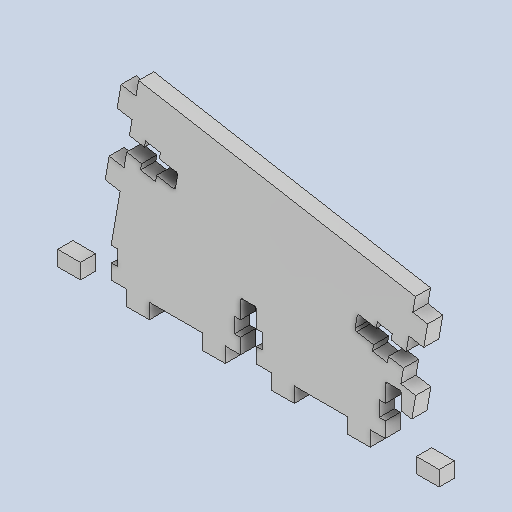
# Autodesk Inventor part: tc_support_down
Saved by Autodesk Inventor 2024.1 (Build 281209000, 209)
## iProperties
Created: 2019-07-16
Part Number: tc_support_down
Material: Acier inoxydable
Document SubType Name: Modeling
Designer: Thibault
Density: 8 g/cm^3
Appearance: Semi-poli
extra_height_front: 10,900 mm
extra_height_back: 4,367 mm
tc_base_support_dist: 37,050 mm
tc_anchor_dist: 19,100 mm
Author: Thibault
Autodesk Inventor part; units mm, degrees
ref_plane "YZ Plane" through (0, 0, 0) normal (1, 0, 0) x (0, 1, 0)
ref_plane "XZ Plane" through (0, 0, 0) normal (0, 1, 0) x (-1, 0, 0)
ref_plane "XY Plane" through (0, 0, 0) normal (0, 0, 1) x (1, 0, 0)
sketch "Anchor (nut side)" plane through (0, 0, 0) normal (0, 0, 1) x (1, 0, 0)
  line L0 (11.1, 0) -> (9.1, 0)
  line L1 (9.1, 0) -> (9.1, -2)
  line L2 (9.1, -2) -> (9.9, -2)
  line L3 (9.9, -2) -> (9.9, -4)
  line L4 (6.2, -4) -> (6.2, -2)
  line L5 (6.2, -2) -> (7, -2)
  line L6 (7, -2) -> (7, 0)
  line L7 (7, 0) -> (5, 0)
  line L8 (2, 0) -> (2, 2)
  line L9 (2, 0) -> (3, 0) construction
  line L10 (2, 2) -> (5, 2)
  line L11 (5, 2) -> (5, 0)
  line L12 (11.1, 0) -> (11.1, 2)
  line L13 (11.1, 2) -> (14.1, 2)
  line L14 (14.1, 2) -> (14.1, 0)
  line L15 (0, 0) -> (2, 0)
  line L16 (14.1, 0) -> (16.1, 0)
  line L17 (6.2, -4) -> (7, -4)
  line L18 (9.9, -4) -> (9.1, -4)
  line L19 (7, -4) -> (7, -6.25)
  line L20 (9.1, -4) -> (9.1, -6.25)
  line L21 (7.25, -6.5) -> (8.05, -6.5)
  arc A0 (7, -6.25) -> (7.25, -6.5) centre (7.25, -6.25) ccw
  arc A1 (8.85, -6.5) -> (9.1, -6.25) centre (8.85, -6.25) ccw
  line L22 (8.05, -6.5) -> (8.85, -6.5)
  line L23 (8.05, -3.8983) -> (8.05, -9.959) construction
  point P0 (9.1321, -0.6227)
  point P1 (7, -6.5)
  point P2 (9.1, -6.5)
  dimension "d3" = 2
  dimension "d7" = 6.1
  dimension "d10" = 2
  dimension "d11" = 2
  dimension "d12" = 0.8
  dimension "d13" = 2
  dimension "d14" = 0.8
  dimension "d15" = 2.1
  dimension "d18" = 2
  dimension "d19" = 0.8
  dimension "d20" = 0.8
  dimension "d21" = 2.5
  dimension "d22" = 2.5
  dimension "d23" = 2.1
  dimension "d38" = 2
  dimension "d39" = 0.25
  dimension "d120" = 3
  measures "d3" distance of point (0, 0) L8.start
  measures "d7" distance of L7.end L0.start
  measures "d10" distance of L0.start L0.end
  measures "d11" distance of L0.end L1.end
  measures "d12" distance of L1.end L2.end
  measures "d13" distance of L2.end L3.end
  measures "d14" distance of L4.end L5.end
  measures "d15" distance of L6.end L0.end
  measures "d18" distance of L14.end point (16.1, 0)
  measures "d19" distance of L4.start L17.end
  measures "d20" distance of L3.end L18.end
  measures "d21" distance of L17.end point (7, -6.5)
  measures "d22" distance of L18.end point (9.1, -6.5)
  measures "d23" distance of L17.end L18.end
  measures "d38" distance of the line from the sketch origin of L10
  measures "d39" radius of A0
  measures "d120" distance of L8.end L10.end
sketch "Anchor (screw side)" plane through (0, 0, 0) normal (0, 0, 1) x (1, 0, 0)
  circle A0 centre (93.8994, 50.2542) radius 1.05
  line L0 (90.8494, 51.2542) -> (87.8494, 51.2542)
  line L1 (87.8494, 51.2542) -> (87.8494, 49.2542)
  line L2 (87.8494, 49.2542) -> (90.8494, 49.2542)
  line L3 (90.8494, 49.2542) -> (90.8494, 51.2542)
  line L4 (99.9494, 51.2542) -> (96.9494, 51.2542)
  line L5 (96.9494, 51.2542) -> (96.9494, 49.2542)
  line L6 (96.9494, 49.2542) -> (99.9494, 49.2542)
  line L7 (99.9494, 49.2542) -> (99.9494, 51.2542)
  line L8 (90.8494, 51.2542) -> (96.9494, 49.2542) construction
  line L9 (96.9494, 51.2542) -> (90.8494, 49.2542) construction
  line L10 (85.8494, 53.2542) -> (101.9494, 53.2542) construction
  line L11 (101.9494, 53.2542) -> (101.9494, 47.2542) construction
  line L12 (101.9494, 47.2542) -> (85.8494, 47.2542) construction
  line L13 (85.8494, 47.2542) -> (85.8494, 53.2542) construction
  point P0 (103.5798, 50.1132)
  dimension "d27" = 2.1
  dimension "d28" = 3
  dimension "d29" = 2
  dimension "slot_distance" = 6.1
  dimension "d34" = 2
  dimension "d35" = 2
  dimension "d36" = 2
  dimension "d37" = 2
  measures "d27" diameter of A0
  measures "d28" distance of L2.end L1.end
  measures "d29" distance of L1.end L0.end
  measures "slot_distance" distance between parallel lines of L5 L3
  measures "d34" distance between parallel lines of L0 L10
  measures "d35" distance between parallel lines of L12 L2
  measures "d36" distance between parallel lines of L11 L7
  measures "d37" distance between parallel lines of L13 L1
derived "shared_parameters.ipt"
sketch "Esquisse2" plane through (0, 0, 0) normal (0, 0, 1) x (1, 0, 0)
  line L0 (-1.0016, 15.2398) -> (1.9984, 15.2398)
  line L1 (18.0984, 15.2398) -> (21.0984, 15.2398)
  line L2 (-17.1016, 15.2398) -> (-8.7624, 15.2398)
  line L3 (37.1984, 15.2398) -> (28.8592, 15.2398)
  line L4 (-8.7624, 15.2398) -> (-7.2169, 24.0046)
  line L5 (-4.4212, 39.86) -> (32.066, 33.4264)
  line L6 (29.2702, 17.571) -> (28.8592, 15.2398)
  line L7 (-12.1016, 15.2398) -> (-10.1016, 15.2398)
  line L8 (-10.1016, 15.2398) -> (-10.1016, 17.2398)
  line L9 (-10.1016, 17.2398) -> (-10.9016, 17.2398)
  line L10 (-10.9016, 17.2398) -> (-10.9016, 19.2398)
  line L11 (-7.2016, 19.2398) -> (-7.2016, 17.2398)
  line L12 (-7.2016, 17.2398) -> (-8.0016, 17.2398)
  line L13 (-8.0016, 17.2398) -> (-8.0016, 15.2398)
  line L14 (-8.0016, 15.2398) -> (-6.0016, 15.2398)
  line L15 (-3.0016, 15.2398) -> (-3.0016, 13.2398)
  line L16 (-3.0016, 15.2398) -> (-4.0016, 15.2398) construction
  line L17 (-3.0016, 13.2398) -> (-6.0016, 13.2398)
  line L18 (-6.0016, 13.2398) -> (-6.0016, 15.2398)
  line L19 (-12.1016, 15.2398) -> (-12.1016, 13.2398)
  line L20 (-12.1016, 13.2398) -> (-15.1016, 13.2398)
  line L21 (-15.1016, 13.2398) -> (-15.1016, 15.2398)
  line L22 (-1.0016, 15.2398) -> (-3.0016, 15.2398)
  line L23 (-15.1016, 15.2398) -> (-17.1016, 15.2398)
  line L24 (-7.2016, 19.2398) -> (-8.0016, 19.2398)
  line L25 (-10.9016, 19.2398) -> (-10.1016, 19.2398)
  line L26 (-8.0016, 19.2398) -> (-8.0016, 21.4898)
  line L27 (-10.1016, 19.2398) -> (-10.1016, 21.4898)
  line L28 (-8.2516, 21.7398) -> (-9.0516, 21.7398)
  arc A0 (-8.0016, 21.4898) -> (-8.2516, 21.7398) centre (-8.2516, 21.4898) ccw
  arc A1 (-9.8516, 21.7398) -> (-10.1016, 21.4898) centre (-9.8516, 21.4898) ccw
  line L29 (-9.0516, 21.7398) -> (-9.8516, 21.7398)
  line L30 (-9.0516, 19.1381) -> (-9.0516, 25.1989) construction
  line L31 (6.9984, 15.2398) -> (8.9984, 15.2398)
  line L32 (8.9984, 15.2398) -> (8.9984, 17.2398)
  line L33 (8.9984, 17.2398) -> (8.1984, 17.2398)
  line L34 (8.1984, 17.2398) -> (8.1984, 19.2398)
  line L35 (11.8984, 19.2398) -> (11.8984, 17.2398)
  line L36 (11.8984, 17.2398) -> (11.0984, 17.2398)
  line L37 (11.0984, 17.2398) -> (11.0984, 15.2398)
  line L38 (11.0984, 15.2398) -> (13.0984, 15.2398)
  line L39 (16.0984, 15.2398) -> (16.0984, 13.2398)
  line L40 (16.0984, 15.2398) -> (15.0984, 15.2398) construction
  line L41 (16.0984, 13.2398) -> (13.0984, 13.2398)
  line L42 (13.0984, 13.2398) -> (13.0984, 15.2398)
  line L43 (6.9984, 15.2398) -> (6.9984, 13.2398)
  line L44 (6.9984, 13.2398) -> (3.9984, 13.2398)
  line L45 (3.9984, 13.2398) -> (3.9984, 15.2398)
  line L46 (18.0984, 15.2398) -> (16.0984, 15.2398)
  line L47 (3.9984, 15.2398) -> (1.9984, 15.2398)
  line L48 (11.8984, 19.2398) -> (11.0984, 19.2398)
  line L49 (8.1984, 19.2398) -> (8.9984, 19.2398)
  line L50 (11.0984, 19.2398) -> (11.0984, 21.4898)
  line L51 (8.9984, 19.2398) -> (8.9984, 21.4898)
  line L52 (10.8484, 21.7398) -> (10.0484, 21.7398)
  arc A2 (11.0984, 21.4898) -> (10.8484, 21.7398) centre (10.8484, 21.4898) ccw
  arc A3 (9.2484, 21.7398) -> (8.9984, 21.4898) centre (9.2484, 21.4898) ccw
  line L53 (10.0484, 21.7398) -> (9.2484, 21.7398)
  line L54 (10.0484, 19.1381) -> (10.0484, 25.1989) construction
  line L55 (26.0984, 15.2398) -> (28.0984, 15.2398)
  line L56 (28.0984, 15.2398) -> (28.0984, 17.2398)
  line L57 (28.0984, 17.2398) -> (27.2984, 17.2398)
  line L58 (27.2984, 17.2398) -> (27.2984, 19.2398)
  line L59 (30.9984, 19.2398) -> (30.9984, 17.2398)
  line L60 (30.9984, 17.2398) -> (30.1984, 17.2398)
  line L61 (30.1984, 17.2398) -> (30.1984, 15.2398)
  line L62 (30.1984, 15.2398) -> (32.1984, 15.2398)
  line L63 (35.1984, 15.2398) -> (35.1984, 13.2398)
  line L64 (35.1984, 15.2398) -> (34.1984, 15.2398) construction
  line L65 (35.1984, 13.2398) -> (32.1984, 13.2398)
  line L66 (32.1984, 13.2398) -> (32.1984, 15.2398)
  line L67 (26.0984, 15.2398) -> (26.0984, 13.2398)
  line L68 (26.0984, 13.2398) -> (23.0984, 13.2398)
  line L69 (23.0984, 13.2398) -> (23.0984, 15.2398)
  line L70 (37.1984, 15.2398) -> (35.1984, 15.2398)
  line L71 (23.0984, 15.2398) -> (21.0984, 15.2398)
  line L72 (30.9984, 19.2398) -> (30.1984, 19.2398)
  line L73 (27.2984, 19.2398) -> (28.0984, 19.2398)
  line L74 (30.1984, 19.2398) -> (30.1984, 21.4898)
  line L75 (28.0984, 19.2398) -> (28.0984, 21.4898)
  line L76 (29.9484, 21.7398) -> (29.1484, 21.7398)
  arc A4 (30.1984, 21.4898) -> (29.9484, 21.7398) centre (29.9484, 21.4898) ccw
  arc A5 (28.3484, 21.7398) -> (28.0984, 21.4898) centre (28.3484, 21.4898) ccw
  line L77 (29.1484, 21.7398) -> (28.3484, 21.7398)
  line L78 (29.1484, 19.1381) -> (29.1484, 25.1989) construction
  line L79 (-5.2894, 34.936) -> (-5.6367, 32.9664)
  line L80 (-5.6367, 32.9664) -> (-3.6671, 32.6191)
  line L81 (-3.6671, 32.6191) -> (-3.5282, 33.4069)
  line L82 (-3.5282, 33.4069) -> (-1.5586, 33.0596)
  line L83 (-2.201, 29.4158) -> (-4.1707, 29.7631)
  line L84 (-4.1707, 29.7631) -> (-4.0317, 30.551)
  line L85 (-4.0317, 30.551) -> (-6.0014, 30.8983)
  line L86 (-6.0014, 30.8983) -> (-6.3487, 28.9287)
  line L87 (-6.8696, 25.9742) -> (-8.8392, 26.3215)
  line L88 (-6.8696, 25.9742) -> (-6.696, 26.9591) construction
  line L89 (-8.8392, 26.3215) -> (-8.3183, 29.276)
  line L90 (-8.3183, 29.276) -> (-6.3487, 28.9287)
  line L91 (-5.2894, 34.936) -> (-7.259, 35.2833)
  line L92 (-7.259, 35.2833) -> (-6.7381, 38.2377)
  line L93 (-6.7381, 38.2377) -> (-4.7685, 37.8904)
  line L94 (-7.2169, 24.0046) -> (-6.8696, 25.9742)
  line L95 (-4.7685, 37.8904) -> (-4.4212, 39.86)
  line L96 (-2.201, 29.4158) -> (-2.0621, 30.2037)
  line L97 (-1.5586, 33.0596) -> (-1.6975, 32.2718)
  line L98 (-2.0621, 30.2037) -> (0.1537, 29.813)
  line L99 (-1.6975, 32.2718) -> (0.5183, 31.8811)
  line L100 (0.4433, 30.0158) -> (0.5822, 30.8036)
  arc A6 (0.1537, 29.813) -> (0.4433, 30.0158) centre (0.1971, 30.0592) ccw
  arc A7 (0.7211, 31.5915) -> (0.5183, 31.8811) centre (0.4749, 31.6349) ccw
  line L101 (0.5822, 30.8036) -> (0.7211, 31.5915)
  line L102 (-1.98, 31.2554) -> (3.9887, 30.203) construction
  line L103 (30.1385, 22.495) -> (30.4858, 24.4646)
  line L104 (30.4858, 24.4646) -> (28.5162, 24.8119)
  line L105 (28.5162, 24.8119) -> (28.3772, 24.0241)
  line L106 (28.3772, 24.0241) -> (26.4076, 24.3714)
  line L107 (27.0501, 28.0152) -> (29.0197, 27.6679)
  line L108 (29.0197, 27.6679) -> (28.8808, 26.88)
  line L109 (28.8808, 26.88) -> (30.8504, 26.5327)
  line L110 (30.8504, 26.5327) -> (31.1977, 28.5023)
  line L111 (31.7187, 31.4568) -> (33.6883, 31.1095)
  line L112 (31.7187, 31.4568) -> (31.545, 30.4719) construction
  line L113 (33.6883, 31.1095) -> (33.1673, 28.155)
  line L114 (33.1673, 28.155) -> (31.1977, 28.5023)
  line L115 (30.1385, 22.495) -> (32.1081, 22.1477)
  line L116 (32.1081, 22.1477) -> (31.5871, 19.1933)
  line L117 (31.5871, 19.1933) -> (29.6175, 19.5406)
  line L118 (32.066, 33.4264) -> (31.7187, 31.4568)
  line L119 (29.6175, 19.5406) -> (29.2702, 17.571)
  line L120 (27.0501, 28.0152) -> (26.9112, 27.2273)
  line L121 (26.4076, 24.3714) -> (26.5465, 25.1592)
  line L122 (26.9112, 27.2273) -> (24.6954, 27.618)
  line L123 (26.5465, 25.1592) -> (24.3307, 25.5499)
  line L124 (24.4058, 27.4152) -> (24.2668, 26.6274)
  arc A8 (24.6954, 27.618) -> (24.4058, 27.4152) centre (24.652, 27.3718) ccw
  arc A9 (24.1279, 25.8395) -> (24.3307, 25.5499) centre (24.3741, 25.7961) ccw
  line L125 (24.2668, 26.6274) -> (24.1279, 25.8395)
  line L126 (26.8291, 26.1756) -> (20.8604, 27.228) construction
  point P0 (0, 0)
  point P1 (38.5311, 15.2398)
  point P2 (-4.4212, 39.86)
  point P3 (-17.8871, 8.2607)
  point P4 (38.6612, 14.1706)
  point P5 (-17.9917, 8.6071)
  point P6 (-15.1016, 15.2398)
  point P7 (32.1984, 15.2398)
  point P8 (-8.0016, 19.5544)
  point P9 (30.1984, 19.4382)
  point P10 (30.1984, 15.2398)
  dimension "d1" = 7
  dimension "d2" = 7
  dimension "tc_anchor_dist" = 19.1
  dimension "height" = 25
  dimension "d41" = 37.05
  dimension "d44" = 80
  dimension "extra_height_front" = 10.9
  dimension "extra_height_back" = 4.3671
  constraints: 14 end point, 5 horizontal, 1 collinear, 14 other
  measures "d41" distance of L5.end L5.start
  measures "d44" angle of L2 L4
extrude "Extrusion1" add sketch "Esquisse2" along normal blind 2 contours L22 L15 L17 L18 L14 L13 L12 L11 L24 L26 L4 L94 L87 L89 L90 L86 L85 L84 L83 L96 L98 A6 L100 L101 A7 L99 L97 L82 L81 L80 L79 L91 L92 L93 L95 L5 L118 L111 L113 L114 L110 L109 L108 L107 L120 L122 A8 L124 L125 A9 L123 L121 L106 L105 L104 L103 L115 L116 L117 L74 A4 L76 L77 A5 L75 L73 L58 L57 L56 L55 L67 L68 L69 L71 L1 L46 L39 L41 L42 L38 L37 L36 L35 L48 L50 A2 L52 L53 A3 L51 L49 L34 L33 L32 L31 L43 L44 L45 L47 L0 | L2 L19 L20 L21 | L63 L65 L66 L3
equation "\"d41\" = tc_base_support_dist"
equation "\"d31\" = sheet_thickness"
equation "\"tc_base_support_dist\" = 37.05"
equation "\"sheet_thickness\" = 2"
